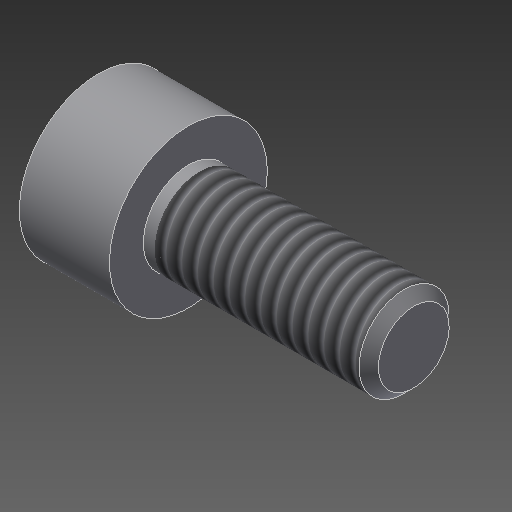
# Autodesk Inventor part: CBM4-10
Saved by Autodesk Inventor 2021.1 (Build 251245010, 245A)
## iProperties
Created: 2010-03-07
Part Number: CBM4-10
Catalog Web Link: www.cadenas.de
Document SubType Name: Modeling
Density: 1 g/cm^3
Material: MISUMI
Appearance: 既定
Category: PARTsolutions
NB: CBM4-10
NN: CBM
NT: Hexagon Socket Head Cap Screws - Bright Chromate
NBSYN: $PN.
LINA: CBM4-10
PN: CBM4-10
MAT: 4137 Steel
ST: Bright Chromate
M: 4
L: 10
LL: Full Thread
L1: 20.000
TYPE: CBM
M1: 4
L0: 6,8,10,12,15,18,20,25,30,35,40
NDM: 4.000
KDM: 3.140
MP: 4x0.7
P: 0.700
A: 7.0
E: 4.0
B: 3.0
KT: DUMMY
PSOL_IDENT_0: {\\10.0.0.149\dplatte\cadenas\23d-libs\misumi\metric\27_screws_nuts\cbm.prj},154 {VTYP=3D},{NB=CBM4-
PSOL_IDENT_1: 10},{LINA=CBM4-10},{NN=CBM},{DATE=02.04.2009 09:44:58},{GEOMDATE=25.02.2009 11:10:00},{VERSION=},{LI
PSOL_IDENT_2: NEID=20},{LINESUBID=-1},{WBVAR=L}  {NB=CBM4-10},{LINA=CBM4-10},{KT=DUMMY},{IDNR=},{PN=CBM4-10},{MAT=
PSOL_IDENT_3: 4137 Steel},{ST=Bright Chromate},{M=4},{L=10},{LL=Full Thread},{L1=20},{TYPE=CBM},{M1=4},{L0=6,8,10,
PSOL_IDENT_4: 12,15,18,20,25,30,35,40},{NDM=4},{KDM=3.139931},{MP=4x0.7},{P=0.7},{A=7.0},{E=4.0},{B=3.0}
Title: 六角穴付ボルト
Comments: Hexagon Socket Head Cap Screws - Bright Chromate
Autodesk Inventor part; units mm, degrees
sketch "Sketch_1" plane through (0, 0, 0) normal (0, 0, 1) x (1, 0, 0)
  line L0 (10, 0) -> (-4, 0)
  line L1 (-4, 0) -> (-4, 3.5)
  line L2 (-4, 3.5) -> (0, 3.5)
  line L3 (0, 3.5) -> (0, 2)
  line L4 (0, 2) -> (9.5705, 2)
  line L5 (9.5705, 2) -> (10, 1.5705)
  line L6 (10, 1.5705) -> (10, 0)
  line L7 (10, 0) -> (-4, 0)
  constraints: 16 end point
revolve "Revolution1" add sketch "Sketch_1" angle 360 about axis through (10, 0, 0) along (1, 0, 0)
thread "Thread1" size "M4x0.7" class "6g" standard "ISO Metric profile" length 9.5 offset 0.5
sketch "Sketch_4" plane through (0, 0, 0) normal (0, 0, 1) x (1, 0, 0)
  line L0 (-1.5981, 0) -> (-4, 0)
  line L1 (-4, 0) -> (-4, 1.5)
  line L2 (-4, 1.5) -> (-2, 1.5)
  line L3 (-2, 1.5) -> (-1.5981, 0)
  line L4 (-1.5981, 0) -> (-4, 0)
  constraints: 10 end point
revolve "Revolution2" cut sketch "Sketch_4" angle 360 about axis through (-1.5981, 0, 0) along (1, 0, 0)
sketch "Sketch_3" plane through (-4, 0, 0) normal (1, 0, 0) x (0, 0, -1)
  line L0 (-1.5, 0.866) -> (-1.5, -0.866)
  line L1 (-1.5, -0.866) -> (0, -1.7321)
  line L2 (0, -1.7321) -> (1.5, -0.866)
  line L3 (1.5, -0.866) -> (1.5, 0.866)
  line L4 (1.5, 0.866) -> (0, 1.7321)
  line L5 (0, 1.7321) -> (-1.5, 0.866)
  constraints: 12 end point
extrude "Extrusion1" cut sketch "Sketch_3" along normal blind 2
ref_plane "bolt_XY" through (0, 0, 0) normal (1, 0, 0) x (0, 0, -1)
ref_plane "bolt_YZ" through (0, 0, 0) normal (0, 0, -1) x (0, 1, 0)
ref_plane "bolt_ZX" through (0, 0, 0) normal (0, 1, 0) x (1, 0, 0)
ref_plane "nut_XY" through (10, 0, 0) normal (1, 0, 0) x (0, 0, -1)
ref_plane "nut_YZ" through (10, 0, 0) normal (0, 0, -1) x (0, 1, 0)
ref_plane "nut_ZX" through (10, 0, 0) normal (0, 1, 0) x (1, 0, 0)
